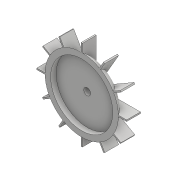
# Autodesk Inventor part: SnackClock_interior_final
Saved by Autodesk Inventor 2018 (Build 220112000, 112)
## iProperties
Created: 2018-02-19
Part Number: SnackClock_interior_final
Material: Generic
Document SubType Name: Modeling
Designer: Katrina
Density: 1 g/cm^3
Appearance: Default
Mass: 10.7451 g
Surface Area: 84.3888 cm^2
Volume: 10.7451 cm^3
Author: Katrina
Autodesk Inventor part; units mm, degrees
ref_plane "YZ Plane" through (0, 0, 0) normal (1, 0, 0) x (0, 1, 0)
ref_plane "XZ Plane" through (0, 0, 0) normal (0, 1, 0) x (-1, 0, 0)
ref_plane "XY Plane" through (0, 0, 0) normal (0, 0, 1) x (1, 0, 0)
sketch "Sketch1" plane through (0, 0, 0) normal (0, 1, 0) x (-1, 0, 0)
  circle A0 centre (0, 0) radius 26.5
  dimension "d0" = 53
  constraints: 1 centre point, 1 coincident
  measures "d0" diameter of A0
extrude "Extrusion1" add sketch "Sketch1" along normal blind 12
fillet "Fillet1" radius 26.5 1 edges at (26.5, 12, 0)
sketch "Sketch3" plane through (0, 0, 0) normal (0, -1, 0) x (1, 0, 0)
  line L0 (32.5, 0.5) -> (-32.5, 0.5)
  line L1 (-32.5, 0.5) -> (-32.5, -0.5)
  line L2 (-32.5, -0.5) -> (32.5, -0.5)
  line L3 (32.5, -0.5) -> (32.5, 0.5)
  point P0 (0, 0)
  point P1 (32.5, 0)
  point P2 (0, -0.5)
  dimension "d7" = 65
  dimension "d8" = 1
  constraints: 8 end point, 2 midpoint, 2 parallel, 1 horizontal, 1 horizontal alignment, 1 perpendicular, 1 vertical alignment
  measures "d7" distance of L2.end L1.end
  measures "d8" distance of L1.end L0.end
extrude "Extrusion3" add sketch "Sketch3" against normal blind 10
pattern_circular "Circular Pattern1" count 12 over 360 about axis through (0, -10, 0) along (0, 1, 0) of "Extrusion3"
sketch "Sketch2" plane through (0, 0, 0) normal (0, -1, 0) x (1, 0, 0)
  circle A0 centre (0, 0) radius 22.5
  dimension "d3" = 45
  constraints: 1 centre point, 1 coincident
  measures "d3" diameter of A0
extrude "Extrusion2" cut sketch "Sketch2" against normal blind 4
sketch "Sketch4" plane through (0, 12, 0) normal (0, 1, 0) x (1, 0, 0)
  circle A0 centre (0, 0) radius 4.3189 projected
  circle A1 centre (0, 0) radius 2.5
  dimension "d14" = 5
  constraints: 1 centre point, 1 coincident
  measures "d14" diameter of A1
extrude "Extrusion4" cut sketch "Sketch4" against normal through all contours A1
body "Solid1"
